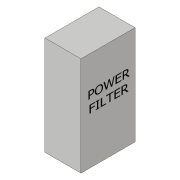
# Autodesk Inventor part: RFI_power_filter
Saved by Autodesk Inventor 2017 (Build 210142000, 142)
## iProperties
Created: 2016-11-14
Part Number: RFI_power_filter
Material: Generic
Document SubType Name: Modeling
Designer: krosie
Density: 1 g/cm^3
Appearance: Default
Author: krosie
Autodesk Inventor part; units mm, degrees
ref_plane "YZ Plane" through (0, 0, 0) normal (1, 0, 0) x (0, 1, 0)
ref_plane "XZ Plane" through (0, 0, 0) normal (0, 1, 0) x (-1, 0, 0)
ref_plane "XY Plane" through (0, 0, 0) normal (0, 0, 1) x (1, 0, 0)
sketch "Sketch1" plane through (0, 0, 0) normal (1, 0, 0) x (0, 1, 0)
  line L0 (0, 90) -> (330, 90)
  line L1 (330, 90) -> (330, -90)
  line L2 (330, -90) -> (0, -90)
  line L3 (0, -90) -> (0, 90)
  line L4 (0, 0) -> (345.997, 0) construction
  dimension "d0" = 330
  dimension "d1" = 180
  constraints: 10 end point, 2 parallel, 2 perpendicular, 1 horizontal, 1 other
  measures "d0" distance of L1.end L2.end
  measures "d1" distance of L0.end L1.end
extrude "Extrusion1" add sketch "Sketch1" along normal blind 120
sketch "Sketch2" plane through (120, 0, 0) normal (1, 0, 0) x (0, 0, -1)
  line L0 (-5.1081, 224.8212) -> (8.9019, 224.8212) construction
  line L1 (8.9019, 224.8212) -> (8.9019, 216.6905) construction
  line L2 (8.9019, 216.6905) -> (-5.1081, 216.6905) construction
  line L3 (-5.1081, 216.6905) -> (-5.1081, 224.8212) construction
  point P0 (0, 0)
  constraints: 2 other
body "Solid1"
